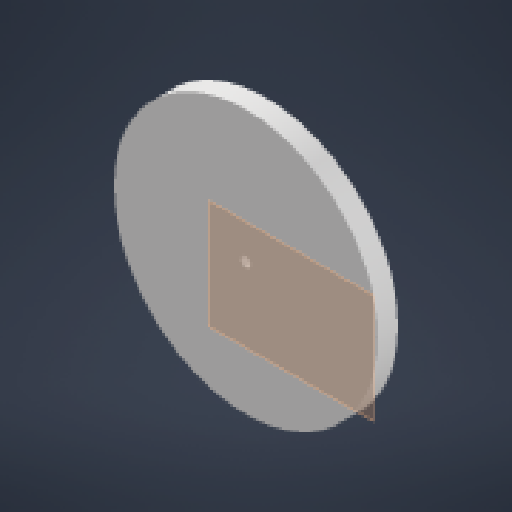
# Autodesk Inventor part: РабОбласть2
Saved by Autodesk Inventor 2026 (Build 300175000, 175)
## iProperties
Created: 2026-04-19
Part Number: РабОбласть2
Material: Стекло
Document SubType Name: Modeling
Designer: Artem Sannikov
Density: 2.18 g/cm^3
Appearance: Бесцветный
Author: Artem Sannikov
Autodesk Inventor part; units mm, degrees
ref_plane "YZ Plane" through (0, 0, 0) normal (1, 0, 0) x (0, 1, 0)
ref_plane "XZ Plane" through (0, 0, 0) normal (0, 1, 0) x (-1, 0, 0)
ref_plane "XY Plane" through (0, 0, 0) normal (0, 0, 1) x (1, 0, 0)
ref_plane "РабПлоскость1" through (0, 0, 0) normal (0, 0, 1) x (1, 0, 0)
sketch "Эскиз1" plane through (0, 0, 0) normal (0, 0, 1) x (1, 0, 0)
  circle A0 centre (-98.3223, 43.4037) radius 11.2136 projected
  circle A1 centre (-98.3223, 43.4037) radius 288.4132
  point P0 (0, 0)
  constraints: 1 centre point, 1 coincident
extrude "Выдавливание1" add sketch "Эскиз1" against normal blind 44.25
